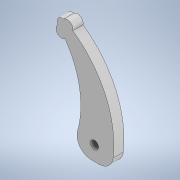
# Autodesk Inventor part: mavac_ruka I guesss
Saved by Autodesk Inventor 2022 (Build 260153000, 153)
## iProperties
Created: 2022-08-25
Part Number: mavac_ruka I guesss
Material: Generic
Document SubType Name: Modeling
Designer: Ruslana Zubareva
Density: 1 g/cm^3
Appearance: Default
Author: Ruslana Zubareva
Autodesk Inventor part; units mm, degrees
ref_plane "YZ Plane" through (0, 0, 0) normal (1, 0, 0) x (0, 1, 0)
ref_plane "XZ Plane" through (0, 0, 0) normal (0, 1, 0) x (-1, 0, 0)
ref_plane "XY Plane" through (0, 0, 0) normal (0, 0, 1) x (1, 0, 0)
sketch "Sketch1" plane through (0, 0, 0) normal (0, 0, 1) x (1, 0, 0)
  arc A0 (6.3455, 7.6592) -> (2.9969, 4.161) centre (5.1207, 5.4798) ccw
  arc A1 (28.9309, -45.2636) -> (10.279, 5.1864) centre (-16.779, -33.4901) ccw
  arc A2 (8.9309, -45.2636) -> (6.4804, -0.2246) centre (-28.4708, -24.7125) ccw
  line L0 (8.9309, -45.2636) -> (28.9309, -45.2636)
  arc A3 (2.9969, 4.161) -> (6.4804, -0.2246) centre (4.7985, 2.0157) ccw
  arc A4 (10.279, 5.1864) -> (5.805, 7.8843) centre (7.5999, 5.8022) ccw
  circle A5 centre (20.9309, -38.1135) radius 2
  point P0 (0, 0)
  dimension "d25" = 2.5
  dimension "d32" = 20
  dimension "d50" = 7.1502
  dimension "d51" = 8
  constraints: 12 point on circle, 6 centre point, 2 end point, 1 horizontal, 1 tangent
  measures "d25" radius of A0
  measures "d32" distance of L0.start L0.end
  measures "d50" distance from line of L0 A5.centre
  measures "d51" horizontal distance of L0.end A5.centre
extrude "Extrusion4" add sketch "Sketch1" along normal blind 5
fillet "Fillet3" radius 7 2 edges at (8.9309, -45.2636, 2.5) (28.9309, -45.2636, 2.5)
body "Solid2"
